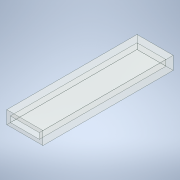
# Autodesk Inventor part: 2mmCuvette
Saved by Autodesk Inventor 2022 (Build 260153000, 153)
## iProperties
Created: 2021-01-23
Part Number: 2mmCuvette
Material: Glass
Document SubType Name: Modeling
Designer: wilso
Density: 2.18 g/cm^3
Appearance: Clear
Author: wilso
Autodesk Inventor part; units mm, degrees
ref_plane "YZ Plane" through (0, 0, 0) normal (1, 0, 0) x (0, 1, 0)
ref_plane "XZ Plane" through (0, 0, 0) normal (0, 1, 0) x (-1, 0, 0)
ref_plane "XY Plane" through (0, 0, 0) normal (0, 0, 1) x (1, 0, 0)
sketch "Sketch1" plane through (0, 0, 0) normal (0, 0, 1) x (1, 0, 0)
  line L0 (0, 0) -> (12.5, 0)
  line L1 (12.5, 0) -> (12.5, 4.5)
  line L2 (12.5, 4.5) -> (0, 4.5)
  line L3 (0, 4.5) -> (0, 0)
  dimension "d0" = 12.5
  dimension "d1" = 4.5
  constraints: 8 end point, 2 parallel, 1 horizontal, 1 perpendicular
  measures "d0" distance of L2.end L1.end
  measures "d1" distance of L1.end L0.end
extrude "Extrusion1" add sketch "Sketch1" along normal blind 45
sketch "Sketch2" plane through (0, 0, 45) normal (0, 0, 1) x (1, 0, 0)
  line L0 (1.25, 1.25) -> (11.25, 1.25)
  line L1 (11.25, 1.25) -> (11.25, 3.25)
  line L2 (11.25, 3.25) -> (1.25, 3.25)
  line L3 (1.25, 3.25) -> (1.25, 1.25)
  line L4 (12.5, 4.5) -> (0, 4.5) projected
  line L5 (0, 4.5) -> (0, 0) projected
  dimension "d4" = 10
  dimension "d5" = 2
  dimension "d6" = 1.25
  dimension "d7" = 1.25
  constraints: 8 end point, 2 parallel, 1 horizontal, 1 perpendicular
  measures "d4" distance of L2.end L1.end
  measures "d5" distance of L1.end L0.end
  measures "d6" distance between parallel lines of L4 L2
  measures "d7" distance between parallel lines of L5 L3
extrude "Extrusion2" cut sketch "Sketch2" against normal blind 43.75
body "Solid1"
